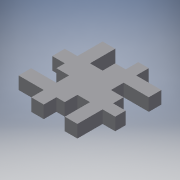
# Autodesk Inventor part: Part4
Saved by Autodesk Inventor 2018 (Build 220112000, 112)
## iProperties
Created: 2018-04-20
Part Number: Part4
Material: Generic
Document SubType Name: Modeling
Designer: Administrator
Density: 1 g/cm^3
Appearance: Default
Author: Administrator
Autodesk Inventor part; units mm, degrees
ref_plane "YZ Plane" through (0, 0, 0) normal (1, 0, 0) x (0, 1, 0)
ref_plane "XZ Plane" through (0, 0, 0) normal (0, 1, 0) x (-1, 0, 0)
ref_plane "XY Plane" through (0, 0, 0) normal (0, 0, 1) x (1, 0, 0)
sketch "Sketch1" plane through (0, 0, 0) normal (0, 1, 0) x (-1, 0, 0)
  line L0 (0, 0) -> (-31.75, 0)
  line L1 (-31.75, 0) -> (-31.75, -31.75)
  line L2 (-31.75, -31.75) -> (0, -31.75)
  line L3 (0, -31.75) -> (0, 0)
  dimension "d0" = 31.75
  dimension "d1" = 31.75
  constraints: 8 end point, 2 parallel, 1 horizontal, 1 perpendicular
  measures "d0" distance between parallel lines of L2 L0
  measures "d1" distance between parallel lines of L1 L3
extrude "Extrusion1" add sketch "Sketch1" along normal blind 4.7625
sketch "Sketch4" plane through (0, 4.7625, 0) normal (0, 1, 0) x (1, 0, 0)
  line L0 (0, 0) -> (9.525, 0)
  line L1 (9.525, 0) -> (9.525, 4.7625)
  line L2 (9.525, 4.7625) -> (0, 4.7625)
  line L3 (0, 4.7625) -> (0, 0)
  line L4 (0, 31.75) -> (0, 0) projected
  line L5 (0, 31.75) -> (4.7625, 31.75)
  line L6 (4.7625, 31.75) -> (4.7625, 22.225)
  line L7 (4.7625, 22.225) -> (0, 22.225)
  line L8 (0, 22.225) -> (0, 31.75)
  line L9 (0, 9.525) -> (4.7625, 9.525)
  line L10 (4.7625, 9.525) -> (4.7625, 17.4625)
  line L11 (4.7625, 17.4625) -> (0, 17.4625)
  line L12 (0, 17.4625) -> (0, 9.525)
  line L13 (0, 0) -> (31.75, 0) projected
  line L14 (14.2875, 0) -> (22.225, 0)
  line L15 (22.225, 0) -> (22.225, 4.7625)
  line L16 (22.225, 4.7625) -> (14.2875, 4.7625)
  line L17 (14.2875, 4.7625) -> (14.2875, 0)
  line L18 (0, 0) -> (31.75, 0) projected
  line L19 (31.75, 0) -> (26.9875, 0)
  line L20 (26.9875, 0) -> (26.9875, 9.525)
  line L21 (26.9875, 9.525) -> (31.75, 9.525)
  line L22 (31.75, 9.525) -> (31.75, 0)
  line L23 (31.75, 0) -> (31.75, 31.75) projected
  line L24 (31.75, 13.4937) -> (26.9875, 13.4937)
  line L25 (26.9875, 13.4937) -> (26.9875, 22.225)
  line L26 (26.9875, 22.225) -> (31.75, 22.225)
  line L27 (31.75, 22.225) -> (31.75, 13.4937)
  line L28 (31.75, 31.75) -> (22.225, 31.75)
  line L29 (22.225, 31.75) -> (22.225, 26.9875)
  line L30 (22.225, 26.9875) -> (31.75, 26.9875)
  line L31 (31.75, 26.9875) -> (31.75, 31.75)
  line L32 (31.75, 31.75) -> (0, 31.75) projected
  line L33 (9.525, 31.75) -> (18.2563, 31.75)
  line L34 (18.2563, 31.75) -> (18.2563, 26.9875)
  line L35 (18.2563, 26.9875) -> (9.525, 26.9875)
  line L36 (9.525, 26.9875) -> (9.525, 31.75)
  dimension "d42" = 9.525
  dimension "d43" = 4.7625
  dimension "d44" = 9.525
  dimension "d46" = 4.7625
  dimension "d48" = 4.7625
  dimension "d49" = 4.7625
  dimension "d50" = 4.7625
  dimension "d51" = 4.7625
  constraints: 64 end point, 16 parallel, 8 horizontal, 8 perpendicular, 6 point on line
  measures "d42" distance between parallel lines of L1 L3
  measures "d43" distance between parallel lines of L2 L0
  measures "d44" distance between parallel lines of L7 L5
  measures "d46" distance between parallel lines of L11 L7
  measures "d48" distance between parallel lines of L9 L2
  measures "d49" distance between parallel lines of L1 L17
  measures "d50" distance between parallel lines of L22 L20
  measures "d51" distance between parallel lines of L15 L20
extrude "Extrusion4" cut sketch "Sketch4" against normal blind 4.7625 contours L3 L2 L1 L0 | L17 L16 L15 L13 | L4 L11 L10 L9 | L20 L21 L22 L13 | L4 L5 L6 L7 | L24 L25 L26 L23 | L32 L34 L35 L36 | L30 L29 L28 L23
sketch "Sketch5" plane through (0, 4.7625, 0) normal (0, 1, 0) x (1, 0, 0)
  line L0 (4.7625, 9.525) -> (9.525, 9.525)
  line L1 (9.525, 9.525) -> (9.525, 14.2875)
  line L2 (9.525, 14.2875) -> (4.7625, 14.2875)
  line L3 (4.7625, 14.2875) -> (4.7625, 9.525)
  line L4 (9.525, 26.9875) -> (18.2563, 26.9875) projected
  line L5 (9.525, 26.9875) -> (14.2875, 26.9875)
  line L6 (14.2875, 26.9875) -> (14.2875, 22.225)
  line L7 (14.2875, 22.225) -> (9.525, 22.225)
  line L8 (9.525, 22.225) -> (9.525, 26.9875)
  line L9 (26.9875, 22.225) -> (26.9875, 13.4937) projected
  line L10 (26.9875, 22.225) -> (22.225, 22.225)
  line L11 (22.225, 22.225) -> (22.225, 17.4625)
  line L12 (22.225, 17.4625) -> (26.9875, 17.4625)
  line L13 (26.9875, 17.4625) -> (26.9875, 22.225)
  line L14 (22.225, 4.7625) -> (14.2875, 4.7625) projected
  line L15 (22.225, 4.7625) -> (17.4625, 4.7625)
  line L16 (17.4625, 4.7625) -> (17.4625, 9.525)
  line L17 (17.4625, 9.525) -> (22.225, 9.525)
  line L18 (22.225, 9.525) -> (22.225, 4.7625)
  point P0 (0, 0)
  dimension "d54" = 4.7625
  dimension "d55" = 4.7625
  dimension "d56" = 4.7625
  dimension "d57" = 4.7625
  dimension "d58" = 4.7625
  dimension "d59" = 4.7625
  dimension "d60" = 4.7625
  dimension "d61" = 4.7625
  constraints: 32 end point, 8 parallel, 4 horizontal, 4 perpendicular
  measures "d54" distance between parallel lines of L1 L3
  measures "d55" distance between parallel lines of L2 L0
  measures "d56" distance between parallel lines of L4 L7
  measures "d57" distance between parallel lines of L6 L8
  measures "d58" distance between parallel lines of L11 L9
  measures "d59" distance between parallel lines of L12 L10
  measures "d60" distance between parallel lines of L17 L15
  measures "d61" distance between parallel lines of L16 L18
extrude "Extrusion5" cut sketch "Sketch5" against normal blind 4.7625
body "Solid1"
